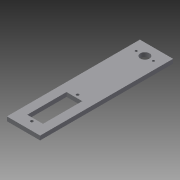
# Autodesk Inventor part: UpperArm
Saved by Autodesk Inventor 2013 (Build 170138000, 138)
## iProperties
Created: 2013-04-21
Part Number: UpperArm
Material: Generic
Document SubType Name: Modeling
Designer: fuji
Density: 1 g/cm^3
Author: fuji
Autodesk Inventor part; units mm, degrees
ref_plane "YZ Plane" through (0, 0, 0) normal (1, 0, 0) x (0, 1, 0)
ref_plane "XZ Plane" through (0, 0, 0) normal (0, 1, 0) x (-1, 0, 0)
ref_plane "XY Plane" through (0, 0, 0) normal (0, 0, 1) x (1, 0, 0)
sketch "Sketch1" plane through (0, 0, 0) normal (0, 1, 0) x (-1, 0, 0)
  line L0 (0, 0) -> (25.4, 0)
  line L1 (25.4, 0) -> (25.4, 101.6)
  line L2 (25.4, 101.6) -> (0, 101.6)
  line L3 (0, 101.6) -> (0, 0)
  circle A0 centre (12.7, 8.89) radius 3.5052
  circle A1 centre (6.1214, 8.89) radius 0.889
  circle A2 centre (19.2786, 8.89) radius 0.889
  line L4 (6.7, 62.71) -> (18.7, 62.71)
  line L5 (18.7, 62.71) -> (18.7, 92.71)
  line L6 (18.7, 92.71) -> (6.7, 92.71)
  line L7 (6.7, 92.71) -> (6.7, 62.71)
  circle A3 centre (12.7, 95.21) radius 1.0541
  circle A4 centre (12.7, 60.21) radius 1.0541
  dimension "d0" = 25.4
  dimension "d1" = 101.6
  dimension "d2" = 7.0104
  dimension "d3" = 8.89
  dimension "d4" = 12.7
  dimension "d5" = 1.778
  dimension "d6" = 1.778
  dimension "d7" = 13.1572
  dimension "d8" = 6.5786
  dimension "d9" = 8.89
  dimension "d10" = 8.89
  dimension "d11" = 12
  dimension "d12" = 30
  dimension "d13" = 8.89
  dimension "d14" = 6.7
  dimension "d15" = 2.1082
  dimension "d16" = 2.1082
  dimension "d17" = 6
  dimension "d18" = 6
  dimension "d19" = 35
  dimension "d20" = 2.5
  constraints: 16 end point, 5 centre point, 4 parallel, 2 horizontal, 2 perpendicular
  measures "d0" distance of L2.end L1.end
  measures "d1" distance of L1.end L0.end
  measures "d2" diameter of A0
  measures "d3" distance from line of A0.centre L0
  measures "d4" distance from line of A0.centre L3
  measures "d5" diameter of A1
  measures "d6" diameter of A2
  measures "d7" distance of A2.centre A1.centre
  measures "d8" distance of A0.centre A1.centre
  measures "d9" distance from line of A1.centre L0
  measures "d10" distance from line of A2.centre L0
  measures "d11" distance of L6.end L5.end
  measures "d12" distance of L5.end L4.end
  measures "d13" distance between parallel lines of L6 L2
  measures "d14" distance between parallel lines of L3 L7
  measures "d15" diameter of A3
  measures "d16" diameter of A4
  measures "d17" distance from line of A4.centre L7
  measures "d18" distance from line of A3.centre L7
  measures "d19" distance of A4.centre A3.centre
  measures "d20" distance from line of A4.centre L4
extrude "Extrusion1" add sketch "Sketch1" along normal blind 3.175
equation "\"d0\" = armWidth"
equation "\"d1\" = armLength"
equation "\"d2\" = hornCenter"
equation "\"d3\" = hornOffset"
equation "\"d4\" = 0.5 * armWidth"
equation "\"d5\" = hornHole"
equation "\"d6\" = hornHole"
equation "\"d7\" = hornDia"
equation "\"d8\" = 0.5 * hornDia"
equation "\"d9\" = hornOffset"
equation "\"d10\" = hornOffset"
equation "\"d11\" = servoWidth"
equation "\"d12\" = servoLength"
equation "\"d13\" = servoOff"
equation "\"d14\" = -0.5 * servoWidth + 0.5 * armWidth"
equation "\"d15\" = servoHole"
equation "\"d16\" = servoHole"
equation "\"d17\" = 0.5 * servoWidth"
equation "\"d18\" = 0.5 * servoWidth"
equation "\"d19\" = servoDist"
equation "\"d20\" = -0.5 * servoLength + 0.5 * servoDist"
equation "\"d21\" = thick"
equation "\"thick\" = 3.175"
equation "\"hornCenter\" = 7.0104"
equation "\"hornDia\" = 13.1572"
equation "\"hornOffset\" = 8.89"
equation "\"hornHole\" = 1.778"
equation "\"servoLength\" = 30"
equation "\"servoWidth\" = 12"
equation "\"servoDist\" = 35"
equation "\"servoHole\" = 2.1082"
equation "\"servoOff\" = 8.89"
equation "\"armWidth\" = 25.4"
equation "\"armLength\" = 101.6"
body "Solid1"
